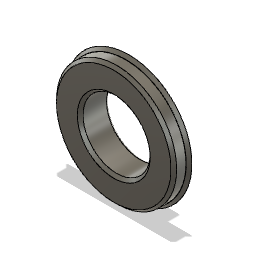
Solder holder axle v1 (Autodesk Fusion 360 design; units mm, degrees)
Autodesk Fusion 360 part; units mm, degrees
sketch "Sketch1" plane through (0, 0, 0) normal (0, 0, 1) x (1, 0, 0)
  circle A0 centre (0, 0) radius 9.5
  dimension "d1" = 19
  constraint coincident A0.centre origin
  measures "d1" diameter of A0
extrude "Extrude1" add sketch "Sketch1" along normal blind 3
sketch "Sketch2" plane through (0, 0, 3) normal (0, 0, 1) x (1, 0, 0)
  circle A0 centre (0, 0) radius 9.5
  circle A1 centre (0, 0) radius 15.5
  dimension "d4" = 31
  constraint concentric A0 A1
  measures "d4" diameter of A1
extrude "Extrude2" add sketch "Sketch2" along normal blind 1 contours A0 | A1
sketch "Sketch3" plane through (0, 0, 4) normal (0, 0, 1) x (1, 0, 0)
  circle A0 centre (0, 0) radius 15.5
  circle A1 centre (0, 0) radius 14.75
  dimension "d7" = 29.5
  constraint coincident A0.centre A1.centre
  measures "d7" diameter of A1
extrude "Extrude3" add sketch "Sketch3" along normal blind 3 contours A1
sketch "Sketch4" plane through (0, 0, 0) normal (0, 0, -1) x (-1, 0, 0)
  circle A0 centre (0, 0) radius 9.5
  circle A1 centre (0, 0) radius 8.25
  dimension "d10" = 16.5
  constraint coincident A0.centre A1.centre
  measures "d10" diameter of A1
extrude "Extrude4" cut sketch "Sketch4" against normal through all contours A1
chamfer "Chamfer1" distance 0.7 angle 45 3 edges at (-13.7518, -5.3338, 7) (7.6917, -2.9833, 7) (-14.4511, -5.605, 4)
fillet "Fillet1" radius 0.5 3 edges at (-14.4511, -5.605, 3) (-8.8571, -3.4353, 0) (7.6917, 2.9833, 0)
equation "d10 = 19 mm - 2.5 mm"
